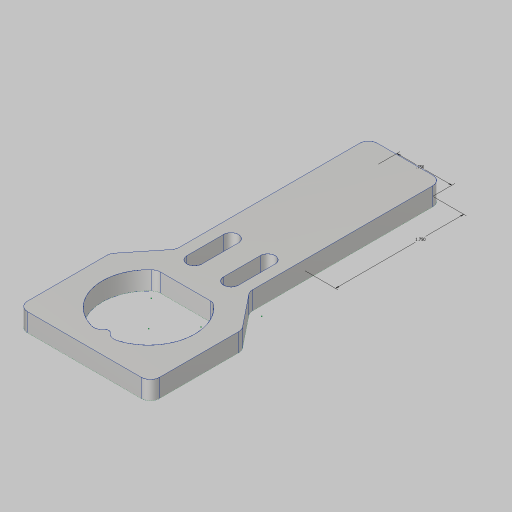
# Autodesk Inventor part: EL2-C-006
Saved by Autodesk Inventor 2023.5 (Build 275446000, 446)
## iProperties
Created: 2025-01-21
Part Number: EL2-C-006
Material: Aluminum 6061
Document SubType Name: Modeling
Designer: slick
Density: 2.7 g/cm^3
Appearance: Aluminum - Flat
Author: slick
Autodesk Inventor part; units mm, degrees
ref_plane "YZ Plane" through (0, 0, 0) normal (1, 0, 0) x (0, 1, 0)
ref_plane "XZ Plane" through (0, 0, 0) normal (0, 1, 0) x (-1, 0, 0)
ref_plane "XY Plane" through (0, 0, 0) normal (0, 0, 1) x (1, 0, 0)
sketch "Sketch1" plane through (0, 0, 0) normal (0, 1, 0) x (-1, 0, 0)
  line L0 (8.89, 0) -> (-8.89, 0) construction
  line L1 (8.89, 1.5875) -> (-8.89, 1.5875)
  line L2 (-8.89, -1.5875) -> (8.89, -1.5875)
  arc A0 (8.89, -1.5875) -> (8.89, 1.5875) centre (8.89, 0) ccw
  arc A1 (-8.89, 1.5875) -> (-8.89, -1.5875) centre (-8.89, 0) ccw
  line L3 (8.89, -5.0038) -> (-8.89, -5.0038) construction
  line L4 (8.89, -3.4163) -> (-8.89, -3.4163)
  line L5 (-8.89, -6.5913) -> (8.89, -6.5913)
  arc A2 (8.89, -6.5913) -> (8.89, -3.4163) centre (8.89, -5.0038) ccw
  arc A3 (-8.89, -3.4163) -> (-8.89, -6.5913) centre (-8.89, -5.0038) ccw
  line L6 (8.89, -10.0076) -> (-8.89, -10.0076) construction
  line L7 (8.89, -8.4201) -> (-8.89, -8.4201)
  line L8 (-8.89, -11.5951) -> (8.89, -11.5951)
  arc A4 (8.89, -11.5951) -> (8.89, -8.4201) centre (8.89, -10.0076) ccw
  arc A5 (-8.89, -8.4201) -> (-8.89, -11.5951) centre (-8.89, -10.0076) ccw
  line L9 (12.7, 58.2549) -> (-12.7, 58.2549)
  line L10 (-12.7, 58.2549) -> (-12.7, -17.9451)
  line L11 (-12.7, -17.9451) -> (12.7, -17.9451)
  line L12 (12.7, -17.9451) -> (12.7, 58.2549)
  line L13 (6.35, 51.9049) -> (-6.35, 51.9049) construction
  arc A6 (8.89, -16.5989) -> (8.89, -13.4239) centre (8.89, -15.0114) ccw
  line L14 (-8.89, -16.5989) -> (8.89, -16.5989)
  arc A7 (-8.89, -13.4239) -> (-8.89, -16.5989) centre (-8.89, -15.0114) ccw
  line L15 (8.89, -13.4239) -> (-8.89, -13.4239)
  arc A8 (-8.89, 6.5913) -> (-8.89, 3.4163) centre (-8.89, 5.0038) ccw
  line L16 (-8.89, 3.4163) -> (8.89, 3.4163)
  line L17 (8.89, 5.0038) -> (-8.89, 5.0038) construction
  line L18 (8.89, 6.5913) -> (-8.89, 6.5913)
  arc A9 (8.89, 3.4163) -> (8.89, 6.5913) centre (8.89, 5.0038) ccw
  arc A10 (-8.89, 11.5951) -> (-8.89, 8.4201) centre (-8.89, 10.0076) ccw
  line L19 (-8.89, 8.4201) -> (8.89, 8.4201)
  line L20 (8.89, 10.0076) -> (-8.89, 10.0076) construction
  line L21 (8.89, 11.5951) -> (-8.89, 11.5951)
  arc A11 (8.89, 8.4201) -> (8.89, 11.5951) centre (8.89, 10.0076) ccw
  arc A12 (-8.89, 16.5989) -> (-8.89, 13.4239) centre (-8.89, 15.0114) ccw
  line L22 (-8.89, 13.4239) -> (8.89, 13.4239)
  line L23 (8.89, 15.0114) -> (-8.89, 15.0114) construction
  line L24 (8.89, 16.5989) -> (-8.89, 16.5989)
  arc A13 (8.89, 13.4239) -> (8.89, 16.5989) centre (8.89, 15.0114) ccw
  point P0 (0, 0)
  point P1 (0, -5.0038)
  point P2 (0, -10.0076)
  point P3 (10.4775, -5.0038)
  point P4 (10.4775, 0)
  point P5 (10.4775, -10.0076)
  point P6 (0, -17.9451)
  point P7 (0, -11.5951)
  point P8 (0, 51.9049)
  point P9 (0, 58.2549)
  point P10 (10.4775, -15.0114)
  point P11 (0, -16.5989)
  point P12 (0, 5.0038)
  point P13 (10.4775, 5.0038)
  point P14 (0, 10.0076)
  point P15 (10.4775, 10.0076)
  point P16 (0, 15.0114)
  point P17 (10.4775, 15.0114)
  dimension "d1" = 17.78
  dimension "d3" = 3.175
  dimension "d4" = 5.0038
  dimension "d5" = 5.0038
  dimension "d8" = 25.4
  dimension "d9" = 76.2
  dimension "d10" = 6.35
  dimension "d11" = 12.7
  dimension "d12" = 6.35
  dimension "d43" = 5.0038
  dimension "d56" = 5.0038
  constraints: 62 end point, 31 point on circle, 14 centre point, 12 tangent, 9 parallel, 7 midpoint, 4 vertical alignment, 3 horizontal, 2 equal radius, 2 vertical, 1 horizontal alignment, 1 perpendicular, 51 other
  measures "d1" distance of L1.start L1.end
  measures "d3" distance between parallel lines of L2 L1
  measures "d4" distance of point (10.477, -5.004) point (10.477, 0)
  measures "d5" distance of point (10.477, -10.008) point (10.477, -5.004)
  measures "d8" distance of L10.end L11.end
  measures "d9" distance of L11.end L9.start
  measures "d10" distance of point (0, -11.595) point (0, -17.945)
  measures "d11" distance of L13.start L13.end
  measures "d12" distance from line of L9 L13.start
  measures "d43" distance of L6.start A6.centre
  measures "d56" distance of L2.start L16.start
extrude "Extrusion1" add sketch "Sketch1" along normal blind 6.35 contours A0 L2 A1 L1 | A2 L5 A3 L4 | A4 L8 A5 L7 | L12 L11 L10 L9 | L14 A7 L15 A6 | L18 A9 L16 A8 | L21 A11 L19 A10 | L24 A13 L22 A12
fillet "Fillet1" radius 3.175 4 edges at (-12.7, 3.175, -17.9451) (12.7, 3.175, -17.9451) (12.7, 3.175, 58.2549) (-12.7, 3.175, 58.2549)
sketch "Sketch2" plane through (0, 6.35, 0) normal (0, 1, 0) x (1, 0, 0)
  line L0 (-6.35, -36.0375) -> (-6.35, -48.7375) construction
  line L1 (-8.9027, -36.0375) -> (-8.9027, -48.7375)
  line L2 (-3.7973, -48.7375) -> (-3.7973, -36.0375)
  arc A0 (-3.7973, -36.0375) -> (-8.9027, -36.0375) centre (-6.35, -36.0375) ccw
  arc A1 (-8.9027, -48.7375) -> (-3.7973, -48.7375) centre (-6.35, -48.7375) ccw
  line L3 (6.35, -36.0375) -> (6.35, -48.7375) construction
  line L4 (3.7973, -36.0375) -> (3.7973, -48.7375)
  line L5 (8.9027, -48.7375) -> (8.9027, -36.0375)
  arc A2 (8.9027, -36.0375) -> (3.7973, -36.0375) centre (6.35, -36.0375) ccw
  arc A3 (3.7973, -48.7375) -> (8.9027, -48.7375) centre (6.35, -48.7375) ccw
  line L6 (-9.525, -58.2549) -> (9.525, -58.2549) projected
  line L7 (9.525, 17.9451) -> (-9.525, 17.9451) projected
  line L8 (-6.35, -42.3875) -> (6.35, -42.3875) construction
  point P0 (0, 0)
  point P1 (0, -42.3875)
  point P2 (0, 17.9451)
  dimension "d23" = 5.1054
  dimension "d24" = 12.7
  dimension "d26" = 60.3326
  dimension "d27" = 12.7
  constraints: 18 end point, 8 point on circle, 8 tangent, 4 centre point, 4 midpoint, 3 parallel, 2 horizontal alignment, 1 equal radius, 1 perpendicular, 1 vertical, 1 vertical alignment
  measures "d23" diameter of A1
  measures "d24" distance of L0.start L0.end
  measures "d26" distance from line of L8.start L7
  measures "d27" distance of L8.start L8.end
extrude "Extrusion2" cut sketch "Sketch2" against normal blind 25.4
sketch "Sketch3" plane through (0, 6.35, 0) normal (0, 1, 0) x (1, 0, 0)
  circle A0 centre (0, -70.9549) radius 16.002
  line L0 (-9.525, -58.2549) -> (9.525, -58.2549) projected
  circle A1 centre (0, -70.9549) radius 19.177
  line L1 (3.7973, -36.0375) -> (3.7973, -48.7375) projected
  arc A2 (3.7973, -48.7375) -> (8.9027, -48.7375) centre (6.35, -48.7375) ccw projected
  line L2 (8.9027, -48.7375) -> (8.9027, -36.0375) projected
  line L3 (-8.9027, -36.0375) -> (-8.9027, -48.7375) projected
  arc A3 (-8.9027, -48.7375) -> (-3.7973, -48.7375) centre (-6.35, -48.7375) ccw projected
  line L4 (-3.7973, -48.7375) -> (-3.7973, -36.0375) projected
  arc A4 (-12.7, -55.0799) -> (-9.525, -58.2549) centre (-9.525, -55.0799) ccw projected
  line L5 (-12.7, -55.0799) -> (-12.7, 14.7701) projected
  arc A5 (-9.525, 17.9451) -> (-12.7, 14.7701) centre (-9.525, 14.7701) ccw projected
  line L6 (-9.525, 17.9451) -> (9.525, 17.9451) projected
  arc A6 (12.7, 14.7701) -> (9.525, 17.9451) centre (9.525, 14.7701) ccw projected
  line L7 (12.7, 14.7701) -> (12.7, -55.0799) projected
  arc A7 (9.525, -58.2549) -> (12.7, -55.0799) centre (9.525, -55.0799) ccw projected
  line L8 (9.525, -58.2549) -> (-9.525, -58.2549) projected
  line L9 (-12.7, -55.0799) -> (-12.7, 14.7701) projected
  arc A8 (-9.525, 17.9451) -> (-12.7, 14.7701) centre (-9.525, 14.7701) ccw projected
  line L10 (-9.525, 17.9451) -> (9.525, 17.9451) projected
  arc A9 (12.7, 14.7701) -> (9.525, 17.9451) centre (9.525, 14.7701) ccw projected
  line L11 (12.7, 14.7701) -> (12.7, -55.0799) projected
  line L12 (9.525, -58.2549) -> (-9.525, -58.2549) projected
  arc A10 (-12.7, -55.0799) -> (-9.525, -58.2549) centre (-9.525, -55.0799) ccw projected
  arc A11 (9.525, -58.2549) -> (12.7, -55.0799) centre (9.525, -55.0799) ccw projected
  line L13 (3.7973, -36.0375) -> (3.7973, -48.7375) projected
  arc A12 (3.7973, -48.7375) -> (8.9027, -48.7375) centre (6.35, -48.7375) ccw projected
  line L14 (8.9027, -48.7375) -> (8.9027, -36.0375) projected
  arc A13 (8.9027, -36.0375) -> (3.7973, -36.0375) centre (6.35, -36.0375) ccw projected
  line L15 (-8.9027, -36.0375) -> (-8.9027, -48.7375) projected
  arc A14 (-8.9027, -48.7375) -> (-3.7973, -48.7375) centre (-6.35, -48.7375) ccw projected
  line L16 (-3.7973, -48.7375) -> (-3.7973, -36.0375) projected
  arc A15 (-3.7973, -36.0375) -> (-8.9027, -36.0375) centre (-6.35, -36.0375) ccw projected
  arc A16 (8.9027, -36.0375) -> (3.7973, -36.0375) centre (6.35, -36.0375) ccw projected
  arc A17 (-3.7973, -36.0375) -> (-8.9027, -36.0375) centre (-6.35, -36.0375) ccw projected
  point P0 (0, 0)
  point P1 (0, -58.2549)
  point P2 (12.433, -56.3543)
  point P3 (9.7268, -58.2485)
  point P4 (-9.7268, -58.2485)
  point P5 (-12.433, -56.3543)
  dimension "d30" = 32.004
  dimension "d31" = 12.7
  dimension "d32" = 3.175
  constraints: 2 centre point, 1 midpoint, 1 vertical alignment
  measures "d30" diameter of A0
  measures "d31" distance from line of L0 A0.centre
  measures "d32" radial gap between concentric circles of A0 A1
extrude "Extrusion3" add sketch "Sketch3" against normal up to surface (6.35 mm away) contours A0 A7 A1 A4 picked at (17.9419, -72.4477)
fillet "Fillet2" radius 3.175 4 edges at (-12.433, 3.175, 56.3543) (12.433, 3.175, 56.3543) (9.7268, 3.175, 58.2485) (-9.7268, 3.175, 58.2485)
sketch "Sketch4" plane through (0, 6.35, 0) normal (0, 1, 0) x (1, 0, 0)
  circle A0 centre (0, -85.8901) radius 1.1811
  arc A1 (-8.5911, -58.2549) -> (-10.7176, -59.0722) centre (-8.5911, -61.4299) ccw projected
  arc A2 (-10.7176, -59.0722) -> (10.7176, -59.0722) centre (0, -70.9549) ccw projected
  arc A3 (10.7176, -59.0722) -> (8.5911, -58.2549) centre (8.5911, -61.4299) ccw projected
  line L0 (8.5911, -58.2549) -> (-8.5911, -58.2549) projected
  arc A4 (12.6992, -55.149) -> (13.6187, -57.4535) centre (15.8735, -55.2182) ccw projected
  arc A5 (-13.6187, -57.4535) -> (13.6187, -57.4535) centre (0, -70.9549) ccw projected
  arc A6 (-13.6187, -57.4535) -> (-12.6992, -55.149) centre (-15.8735, -55.2182) ccw projected
  arc A7 (-12.7, -55.0799) -> (-12.6992, -55.149) centre (-9.525, -55.0799) ccw projected
  line L1 (-12.7, -55.0799) -> (-12.7, 14.7701) projected
  arc A8 (-9.525, 17.9451) -> (-12.7, 14.7701) centre (-9.525, 14.7701) ccw projected
  line L2 (-9.525, 17.9451) -> (9.525, 17.9451) projected
  arc A9 (12.7, 14.7701) -> (9.525, 17.9451) centre (9.525, 14.7701) ccw projected
  line L3 (12.7, 14.7701) -> (12.7, -55.0799) projected
  arc A10 (12.6992, -55.149) -> (12.7, -55.0799) centre (9.525, -55.0799) ccw projected
  line L4 (3.7973, -36.0375) -> (3.7973, -48.7375) projected
  arc A11 (3.7973, -48.7375) -> (8.9027, -48.7375) centre (6.35, -48.7375) ccw projected
  line L5 (8.9027, -48.7375) -> (8.9027, -36.0375) projected
  line L6 (-8.9027, -36.0375) -> (-8.9027, -48.7375) projected
  arc A12 (-8.9027, -48.7375) -> (-3.7973, -48.7375) centre (-6.35, -48.7375) ccw projected
  line L7 (-3.7973, -48.7375) -> (-3.7973, -36.0375) projected
  arc A13 (8.9027, -36.0375) -> (3.7973, -36.0375) centre (6.35, -36.0375) ccw projected
  arc A14 (-3.7973, -36.0375) -> (-8.9027, -36.0375) centre (-6.35, -36.0375) ccw projected
  point P0 (0, 0)
  point P1 (0, -86.9569)
  point P2 (-0.5246, -86.9483)
  point P3 (0.5246, -86.9483)
  dimension "d36" = 2.3622
  dimension "d37" = 1.0668
  constraints: 1 centre point, 1 point on circle
  measures "d36" diameter of A0
  measures "d37" distance of point (0, -86.957) A0.centre
extrude "Extrusion4" add sketch "Sketch4" against normal up to surface (6.35 mm away) contours A0 A2 picked at (-0.0326, -86.2083)
fillet "Fillet3" radius 3.175 2 edges at (-0.5246, 3.175, 86.9483) (0.5246, 3.175, 86.9483)
sketch "Sketch5" plane through (0, 6.35, 0) normal (0, 1, 0) x (1, 0, 0)
  arc A0 (-8.5911, -58.2549) -> (-10.7176, -59.0722) centre (-8.5911, -61.4299) ccw projected
  arc A1 (-10.7176, -59.0722) -> (-4.3651, -86.35) centre (0, -70.9549) ccw projected
  arc A2 (-4.3651, -86.35) -> (-0.9487, -85.1866) centre (-3.499, -83.2954) ccw projected
  arc A3 (0.9487, -85.1866) -> (-0.9487, -85.1866) centre (0, -85.8901) ccw projected
  arc A4 (0.9487, -85.1866) -> (4.3651, -86.35) centre (3.499, -83.2954) ccw projected
  arc A5 (4.3651, -86.35) -> (10.7176, -59.0722) centre (0, -70.9549) ccw projected
  arc A6 (10.7176, -59.0722) -> (8.5911, -58.2549) centre (8.5911, -61.4299) ccw projected
  line L0 (8.5911, -58.2549) -> (-8.5911, -58.2549) projected
  arc A7 (12.6992, -55.149) -> (13.6187, -57.4535) centre (15.8735, -55.2182) ccw projected
  arc A8 (-13.6187, -57.4535) -> (13.6187, -57.4535) centre (0, -70.9549) ccw projected
  arc A9 (-13.6187, -57.4535) -> (-12.6992, -55.149) centre (-15.8735, -55.2182) ccw projected
  arc A10 (-12.7, -55.0799) -> (-12.6992, -55.149) centre (-9.525, -55.0799) ccw construction
  line L1 (-12.7, -55.0799) -> (-12.7, 14.7701) projected
  arc A11 (-9.525, 17.9451) -> (-12.7, 14.7701) centre (-9.525, 14.7701) ccw construction
  line L2 (-9.525, 17.9451) -> (9.525, 17.9451) construction
  arc A12 (12.7, 14.7701) -> (9.525, 17.9451) centre (9.525, 14.7701) ccw construction
  line L3 (12.7, 14.7701) -> (12.7, -55.0799) projected
  arc A13 (12.6992, -55.149) -> (12.7, -55.0799) centre (9.525, -55.0799) ccw construction
  line L4 (3.7973, -36.0375) -> (3.7973, -48.7375) projected
  arc A14 (3.7973, -48.7375) -> (8.9027, -48.7375) centre (6.35, -48.7375) ccw projected
  line L5 (8.9027, -48.7375) -> (8.9027, -36.0375) projected
  line L6 (-8.9027, -36.0375) -> (-8.9027, -48.7375) projected
  arc A15 (-8.9027, -48.7375) -> (-3.7973, -48.7375) centre (-6.35, -48.7375) ccw projected
  line L7 (-3.7973, -48.7375) -> (-3.7973, -36.0375) projected
  line L8 (-12.7, 14.7701) -> (-12.7, -55.0799) construction
  line L9 (12.7, -55.0799) -> (12.7, 14.7701) construction
  arc A16 (8.9027, -36.0375) -> (3.7973, -36.0375) centre (6.35, -36.0375) ccw projected
  arc A17 (-3.7973, -36.0375) -> (-8.9027, -36.0375) centre (-6.35, -36.0375) ccw projected
  line L10 (-22.86, -48.7299) -> (22.86, -48.7299)
  line L11 (22.86, -48.7299) -> (22.86, -93.1799)
  line L12 (22.86, -93.1799) -> (-22.86, -93.1799)
  line L13 (-22.86, -93.1799) -> (-22.86, -48.7299)
  line L14 (-22.86, -48.7299) -> (22.86, -93.1799) construction
  line L15 (22.86, -48.7299) -> (-22.86, -93.1799) construction
  line L16 (-22.86, -61.4299) -> (-12.7, -48.7299)
  line L17 (22.86, -61.4299) -> (12.7, -48.7299)
  point P0 (0, 0)
  point P1 (3.7973, -48.7299)
  point P2 (-3.7973, -48.7299)
  point P3 (-8.9027, -48.7299)
  point P4 (8.9027, -48.7299)
  dimension "d61" = 45.72
  dimension "d62" = 31.75
  dimension "d64" = 44.45
  constraints: 16 end point, 6 point on line, 2 midpoint, 2 parallel, 1 horizontal, 1 horizontal alignment, 1 perpendicular
  measures "d61" distance of L11.end L12.end
  measures "d62" distance of L12.end L16.start
  measures "d64" distance between parallel lines of L12 L10
extrude "Extrusion5" add sketch "Sketch5" against normal up to surface (6.35 mm away) contours L4 A14 L5 L10 L17 L11 L12 L13 L16 L6 A15 L7
fillet "Fillet4" radius 3.175 6 edges at (-22.86, 3.175, 61.4299) (22.86, 3.175, 61.4299) (22.86, 3.175, 93.1799) (-22.86, 3.175, 93.1799) (-12.7, 3.175, 48.7299) (12.7, 3.175, 48.7299)
extrude "Extrusion6" cut sketch "Sketch1" along normal blind 4.445 contours A0 L2 A1 L1 | A2 L5 A3 L4 | A4 L8 A5 L7 | L14 A7 L15 A6 | L18 A9 L16 A8 | L21 A11 L19 A10 | L24 A13 L22 A12
sketch "Sketch7" plane through (0, 0, 0) normal (0, -1, 0) x (1, 0, 0)
  line L0 (9.525, -17.9451) -> (-9.525, -17.9451)
  line L1 (-9.525, -17.9451) -> (-9.525, 26.5049)
  line L2 (-9.525, 26.5049) -> (9.525, 26.5049)
  line L3 (9.525, 26.5049) -> (9.525, -17.9451)
  line L4 (9.525, -17.9451) -> (-9.525, -17.9451) construction
  arc A0 (8.89, 3.4163) -> (8.89, 6.5913) centre (8.89, 5.0038) ccw construction
  line L5 (8.89, 6.5913) -> (-8.89, 6.5913) construction
  arc A1 (-8.89, 6.5913) -> (-8.89, 3.4163) centre (-8.89, 5.0038) ccw construction
  line L6 (-8.89, 3.4163) -> (8.89, 3.4163) construction
  arc A2 (-8.89, -13.4239) -> (-8.89, -16.5989) centre (-8.89, -15.0114) ccw construction
  line L7 (-8.89, -16.5989) -> (8.89, -16.5989) construction
  arc A3 (8.89, -16.5989) -> (8.89, -13.4239) centre (8.89, -15.0114) ccw construction
  line L8 (8.89, -13.4239) -> (-8.89, -13.4239) construction
  line L9 (8.89, 1.5875) -> (-8.89, 1.5875) construction
  arc A4 (-8.89, 1.5875) -> (-8.89, -1.5875) centre (-8.89, 0) ccw construction
  line L10 (-8.89, -1.5875) -> (8.89, -1.5875) construction
  arc A5 (8.89, -1.5875) -> (8.89, 1.5875) centre (8.89, 0) ccw construction
  arc A6 (8.89, 8.4201) -> (8.89, 11.5951) centre (8.89, 10.0076) ccw construction
  line L11 (8.89, 11.5951) -> (-8.89, 11.5951) construction
  arc A7 (-8.89, 11.5951) -> (-8.89, 8.4201) centre (-8.89, 10.0076) ccw construction
  line L12 (-8.89, 8.4201) -> (8.89, 8.4201) construction
  line L13 (8.89, -8.4201) -> (-8.89, -8.4201) construction
  arc A8 (-8.89, -8.4201) -> (-8.89, -11.5951) centre (-8.89, -10.0076) ccw construction
  line L14 (-8.89, -11.5951) -> (8.89, -11.5951) construction
  arc A9 (8.89, -11.5951) -> (8.89, -8.4201) centre (8.89, -10.0076) ccw construction
  line L15 (8.89, -3.4163) -> (-8.89, -3.4163) construction
  arc A10 (-8.89, -3.4163) -> (-8.89, -6.5913) centre (-8.89, -5.0038) ccw construction
  line L16 (-8.89, -6.5913) -> (8.89, -6.5913) construction
  arc A11 (8.89, -6.5913) -> (8.89, -3.4163) centre (8.89, -5.0038) ccw construction
  arc A12 (8.89, 13.4239) -> (8.89, 16.5989) centre (8.89, 15.0114) ccw construction
  line L17 (8.89, 16.5989) -> (-8.89, 16.5989) construction
  arc A13 (-8.89, 16.5989) -> (-8.89, 13.4239) centre (-8.89, 15.0114) ccw construction
  line L18 (-8.89, 13.4239) -> (8.89, 13.4239) construction
  arc A14 (22.86, 90.0049) -> (19.685, 93.1799) centre (19.685, 90.0049) ccw construction
  line L19 (22.86, 90.0049) -> (22.86, 62.5436) construction
  arc A15 (22.1643, 60.5602) -> (22.86, 62.5436) centre (19.685, 62.5436) ccw construction
  line L20 (22.1643, 60.5602) -> (13.3957, 49.5996) construction
  arc A16 (13.3957, 49.5996) -> (12.7, 47.6162) centre (15.875, 47.6162) ccw construction
  line L21 (12.7, 47.6162) -> (12.7, -14.7701) construction
  arc A17 (9.525, -17.9451) -> (12.7, -14.7701) centre (9.525, -14.7701) ccw construction
  line L22 (9.525, -17.9451) -> (-9.525, -17.9451) construction
  arc A18 (-12.7, -14.7701) -> (-9.525, -17.9451) centre (-9.525, -14.7701) ccw construction
  line L23 (-12.7, -14.7701) -> (-12.7, 47.6162) construction
  arc A19 (-12.7, 47.6162) -> (-13.3957, 49.5996) centre (-15.875, 47.6162) ccw construction
  line L24 (-13.3957, 49.5996) -> (-22.1643, 60.5602) construction
  arc A20 (-22.86, 62.5436) -> (-22.1643, 60.5602) centre (-19.685, 62.5436) ccw construction
  line L25 (-22.86, 62.5436) -> (-22.86, 90.0049) construction
  arc A21 (-19.685, 93.1799) -> (-22.86, 90.0049) centre (-19.685, 90.0049) ccw construction
  line L26 (-19.685, 93.1799) -> (19.685, 93.1799) construction
  line L27 (3.7973, 48.7375) -> (3.7973, 36.0375) construction
  arc A22 (3.7973, 36.0375) -> (8.9027, 36.0375) centre (6.35, 36.0375) ccw construction
  line L28 (8.9027, 36.0375) -> (8.9027, 48.7375) construction
  arc A23 (8.9027, 48.7375) -> (3.7973, 48.7375) centre (6.35, 48.7375) ccw construction
  line L29 (-8.9027, 48.7375) -> (-8.9027, 36.0375) construction
  arc A24 (-8.9027, 36.0375) -> (-3.7973, 36.0375) centre (-6.35, 36.0375) ccw construction
  line L30 (-3.7973, 36.0375) -> (-3.7973, 48.7375) construction
  arc A25 (-3.7973, 48.7375) -> (-8.9027, 48.7375) centre (-6.35, 48.7375) ccw construction
  arc A26 (-10.7176, 59.0722) -> (-8.5911, 58.2549) centre (-8.5911, 61.4299) ccw construction
  line L31 (-8.5911, 58.2549) -> (8.5911, 58.2549) construction
  arc A27 (8.5911, 58.2549) -> (10.7176, 59.0722) centre (8.5911, 61.4299) ccw construction
  arc A28 (10.7176, 59.0722) -> (4.3651, 86.35) centre (0, 70.9549) ccw construction
  arc A29 (4.3651, 86.35) -> (0.9487, 85.1866) centre (3.499, 83.2954) ccw construction
  arc A30 (-0.9487, 85.1866) -> (0.9487, 85.1866) centre (0, 85.8901) ccw construction
  arc A31 (-0.9487, 85.1866) -> (-4.3651, 86.35) centre (-3.499, 83.2954) ccw construction
  arc A32 (-4.3651, 86.35) -> (-10.7176, 59.0722) centre (0, 70.9549) ccw construction
  point P0 (0, 0)
  point P1 (0, -17.9451)
  point P2 (0, -17.9451)
  dimension "d72" = 19.05
  dimension "d73" = 44.45
  constraints: 8 end point, 3 midpoint, 2 parallel, 1 coincident, 1 horizontal, 1 perpendicular
  measures "d72" distance of L0.start L0.end
  measures "d73" distance of L2.end L0.start
equation "\"d5\" = d4"
equation "\"d43\" = d5"
body "Solid1"
